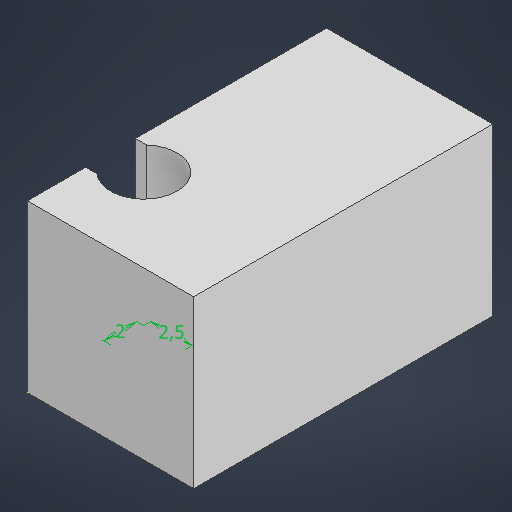
# Autodesk Inventor part: Part9
Saved by Autodesk Inventor 2026.1 (Build 301233020, 233B)
## iProperties
Created: 2025-12-12
Part Number: Part9
Material: Generic
Document SubType Name: Modeling
Designer: alexa
Density: 1 g/cm^3
Appearance: Default
Author: alexa
Autodesk Inventor part; units mm, degrees
ref_plane "YZ Plane" through (0, 0, 0) normal (1, 0, 0) x (0, 1, 0)
ref_plane "XZ Plane" through (0, 0, 0) normal (0, 1, 0) x (-1, 0, 0)
ref_plane "XY Plane" through (0, 0, 0) normal (0, 0, 1) x (1, 0, 0)
sketch "Sketch1" plane through (0, 0, 0) normal (0, 1, 0) x (-1, 0, 0)
  point P0 (0, 0)
sketch "Sketch2" plane through (0, 0, 0) normal (0, 1, 0) x (-1, 0, 0)
  line L0 (0, 0) -> (-5, 0)
  line L1 (-5, 0) -> (-5, -4)
  line L2 (-5, -4) -> (0, -4)
  line L3 (0, -4) -> (0, 0)
  line L4 (0, 0) -> (-10, 0)
  line L5 (-10, 0) -> (-10, -15)
  line L6 (-10, -15) -> (0, -15)
  line L7 (0, -15) -> (0, 0)
  circle A0 centre (-2, -2) radius 2
  line L8 (-5, 0) -> (-2, 0)
  line L9 (-2, 0) -> (-2, -4)
  line L10 (-2, -4) -> (-5, -4)
  line L11 (-5, -4) -> (-5, 0)
  point P0 (0, -2)
  dimension "d0" = 5
  dimension "d1" = 4
  dimension "d2" = 10
  dimension "d3" = 15
  constraints: 24 end point, 6 parallel, 5 horizontal, 3 perpendicular, 1 point on line, 1 vertical, 3 other
  measures "d0" distance of L2.end L1.end
  measures "d1" distance of L1.end L0.end
  measures "d2" distance of L6.end L5.end
  measures "d3" distance of L5.end L4.end
sketch "Sketch3" plane through (0, 0, 0) normal (0, 1, 0) x (-1, 0, 0)
  line L0 (0, 0) -> (0, -4.0004)
  line L1 (0, -4.0004) -> (0, -2.0004)
  line L2 (0, -4.0004) -> (-2.5, -4.0004)
  dimension "d4" = 2
  dimension "d5" = 2.5
  constraints: 6 end point, 1 perpendicular, 1 point on line, 1 vertical
  measures "d4" distance of L0.end L1.end
  measures "d5" distance of L0.end L2.end
extrude "Extrusion1" add sketch "Sketch2" along normal blind 10 contours L3 A0 L0 | A0 L2 L1 L0 | L3 L2 A0 | L1 L2 L7 L6 L5 L4
sketch "Sketch4" plane through (2, 0, 0) normal (0, 0, 1) x (1, 0, 0)
  line L0 (8, 0) -> (8, 10) projected
  line L1 (8, 10) -> (-2, 10)
  line L2 (-2, 10) -> (-2, 0)
  line L3 (-2, 0) -> (8, 0)
  line L4 (8, 0) -> (8, 10)
  constraints: 8 end point, 2 parallel, 1 horizontal, 1 perpendicular
extrude "Extrusion2" add sketch "Sketch4" along normal blind 3
sketch "Sketch5" plane through (0, 0, 0) normal (0, -1, 0) x (1, 0, 0)
  line L0 (0, -15) -> (0, -2) projected
  line L1 (0, -0.3956) -> (0, -3.6044)
  line L2 (0, -3.666) -> (0, -0.334)
  line L3 (0, -2) -> (0, 3) projected
  line L4 (0, -0.334) -> (0, -3.666)
  point P0 (0, 0)
  constraints: 6 end point, 3 midpoint, 2 point on line, 1 collinear
sketch "Sketch6" plane through (0, 0, 0) normal (0, -1, 0) x (1, 0, 0)
  line L0 (0, -15) -> (0, -2) projected
  line L1 (0, -2) -> (0.9417, -2)
  line L2 (0.9417, -2) -> (0.9417, -0.5)
  line L3 (0.9417, -0.5) -> (0, -0.5)
  line L4 (0, -0.5) -> (0, -2)
  circle A0 centre (2, -2) radius 2 projected
  line L5 (0, -2) -> (0.8653, -2)
  line L6 (0.8653, -2) -> (0.8653, -3.5)
  line L7 (0.8653, -3.5) -> (0, -3.5)
  line L8 (0, -3.5) -> (0, -2)
  point P0 (0, 0)
  dimension "d10" = 1.5
  dimension "d11" = 1.5
  constraints: 16 end point, 4 parallel, 2 horizontal, 2 perpendicular, 1 point on circle, 1 point on line
  measures "d10" distance of L2.end L1.end
  measures "d11" distance of L5.end L6.end
extrude "Extrusion3" cut sketch "Sketch6" against normal blind 20 contours L0 A0 L7 | L1 L6 L7 A0
sketch "Sketch7" plane through (0, 0, 0) normal (0, -1, 0) x (1, 0, 0)
  arc A0 (0.6771, -3.5) -> (0, -2) centre (2, -2) ccw projected
  line L0 (0, -2) -> (0.9289, -2)
  line L1 (0.9289, -2) -> (0.9289, -0.5)
  line L2 (0.9289, -0.5) -> (0, -0.5)
  line L3 (0, -0.5) -> (0, -2)
  point P0 (0, 0)
  point P1 (0.6771, -0.5)
  dimension "d14" = 1.5
  constraints: 8 end point, 2 parallel, 1 horizontal, 1 perpendicular
  measures "d14" distance of L1.end L0.end
extrude "Extrusion4" cut sketch "Sketch7" against normal blind 20 contours A0 L3 L2
sketch "Sketch8" plane through (0, 0, 0) normal (0, -1, 0) x (1, 0, 0)
  point P0 (0, 0)
body "Solid1"
